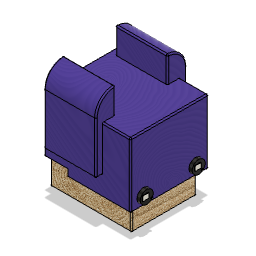
mouth 003 (Autodesk Fusion 360 design; units mm, degrees)
Autodesk Fusion 360 part; units mm, degrees
sketch "Sketch1" plane through (0, 0, 0) normal (0, 0, 1) x (1, 0, 0)
  line L0 (-50.4531, 15) -> (15, 15)
  line L1 (15, 15) -> (15, -10)
  line L2 (15, -10) -> (74.8522, -10)
  line L3 (74.8522, -10) -> (74.8522, -45)
  line L4 (74.8522, -45) -> (-50.4531, -45)
  line L5 (-50.4531, -45) -> (-50.4531, 15)
  constraint horizontal L0
  constraint perpendicular L0 L1
  constraint perpendicular L1 L2
  constraint perpendicular L2 L3
  constraint perpendicular L3 L4
  constraint perpendicular L0 L5
extrude "Extrude1" add sketch "Sketch1" along normal mid plane 100 makes body 1
shell "Shell1" thickness 5 removed faces 3 at (-6.8177, 15, 16.6667) at (15, 6.6667, -16.6667) at (34.9507, -10, -16.6667) on bodies 1
sketch "Sketch2" plane through (0, 0, 0) normal (0, 0, 1) x (1, 0, 0)
  circle A0 centre (0, 0) radius 5
  circle A1 centre (-39.3873, 8.5345) radius 5
  dimension "d4" = 10
  dimension "d5" = 10
  constraint coincident A0.centre origin
  measures "d4" diameter of A0
  measures "d5" diameter of A1
extrude "Extrude2" cut sketch "Sketch2" along normal mid plane 128 bodies 1
sketch "Sketch3" plane through (0, 0, 0) normal (0, 0, 1) x (1, 0, 0)
  line L0 (-50, 90) -> (-50, 0)
  line L1 (-50, 0) -> (-15, 0)
  line L2 (-15, -10) -> (83.2998, -10)
  line L3 (83.2998, -10) -> (83.2998, 90)
  line L4 (83.2998, 90) -> (-50, 90)
  line L5 (-15, 0) -> (-50, 0)
  line L6 (-15, 0) -> (-15, -10)
  constraint vertical L0
  constraint perpendicular L0 L1
  constraint perpendicular L0 L2
  constraint perpendicular L2 L3
  constraint perpendicular L0 L4
  constraint perpendicular L2 L6
extrude "Extrude3" add sketch "Sketch3" along normal mid plane 120 separate body makes body 2
sketch "Sketch4" plane through (-50, 0, 0) normal (-1, 0, 0) x (0, 0, 1)
  line L0 (-60, 0) -> (60, 0)
  line L1 (60, 0) -> (60, 90)
  line L2 (60, 90) -> (-60, 90)
  line L3 (-60, 90) -> (-60, 0)
  line L4 (50, -15) -> (-50, -15)
  line L5 (-50, -15) -> (-50, 20)
  line L6 (-50, 20) -> (50, 20)
  line L7 (50, 20) -> (50, -15)
  constraint horizontal L4
  constraint vertical L5
  constraint horizontal L6
  constraint vertical L7
extrude "Extrude4" cut sketch "Sketch4" against normal blind 120 contours L0 L5 L6 L7 | L0 L4 L5 L7 bodies 2
sketch "Sketch5" plane through (0, 0, 0) normal (0, 0, 1) x (1, 0, 0)
  circle A0 centre (0, 0) radius 5
  circle A1 centre (-39.3873, 8.5345) radius 5
  line L0 (-50.4531, -45) -> (74.8522, -45)
  line L1 (74.8522, -45) -> (74.8522, -10)
  line L2 (74.8522, -10) -> (15, -10)
  line L3 (15, -10) -> (15, 15)
  line L4 (15, 15) -> (-50.4531, 15)
  line L5 (-50.4531, 15) -> (-50.4531, -45)
extrude "Extrude5" add sketch "Sketch5" along normal mid plane 110 contours A1 bodies 2
sketch "Sketch6" plane through (0, 0, 0) normal (0, 0, 1) x (1, 0, 0)
  circle A0 centre (0, 0) radius 5
  circle A1 centre (-39.3873, 8.5345) radius 5
  line L0 (-50.4531, -45) -> (74.8522, -45)
  line L1 (74.8522, -45) -> (74.8522, -10)
  line L2 (74.8522, -10) -> (15, -10)
  line L3 (15, -10) -> (15, 15)
  line L4 (15, 15) -> (-50.4531, 15)
  line L5 (-50.4531, 15) -> (-50.4531, -45)
extrude "Extrude6" add sketch "Sketch6" along normal mid plane 100 separate body contours A0 makes body 3
sketch "Sketch8" plane through (0, 0, 0) normal (0, 0, 1) x (1, 0, 0)
  spline S0 degree 5 poles (0, 10) (-0.4483, 9.945) (-1.2891, 9.7827) (-2.3901, 9.3882) (-3.6145, 8.5811) (-5.0418, 7.1559) (-6.6425, 5.3776) (-8.5424, 3.3303) (-10.5598, 1.1324) (-12.3082, -1.0821) (-13.3437, -3.1875) (-13.2965, -5.0888) (-12.0101, -6.7454) (-9.6761, -8.1935) (-6.7064, -9.5182) (-3.614, -10.8275) (-0.8849, -12.2244) (1.132, -13.782) (2.3779, -15.5123) (3.0801, -17.3558) (3.5942, -19.1894) (4.2991, -20.8317) (5.4495, -22.0404) (7.1257, -22.5462) (9.2752, -22.1244) (11.7289, -20.6623) (14.2302, -18.2134) (16.4761, -14.9495) (18.1594, -11.1255) (19.0092, -7.0404) (18.8343, -2.999) (17.5607, 0.7235) (15.286, 3.9257) (12.2747, 6.494) (8.8775, 8.3796) (5.4706, 9.5855) (3.0039, 10.0369) (1.4007, 10.1128) (0.4483, 10.055) (0, 10) knots 0 0 0 0 0 0 0.028571 0.057143 0.085714 0.114286 0.142857 0.171429 0.2 0.228571 0.257143 0.285714 0.314286 0.342857 0.371429 0.4 0.428571 0.457143 0.485714 0.514286 0.542857 0.571429 0.6 0.628571 0.657143 0.685714 0.714286 0.742857 0.771429 0.8 0.828571 0.857143 0.885714 0.914286 0.942857 0.971429 1 1 1 1 1 1
  point P0 (-7, 5)
  point P1 (-13, -5)
  point P2 (0, -13)
  point P3 (4, -20)
  point P4 (9, -22)
  point P5 (18, -1)
extrude "Extrude8" add sketch "Sketch8" along normal mid plane 88 bodies 3
sketch "Sketch9" plane through (83.2998, 0, 0) normal (1, 0, 0) x (0, 0, -1)
  line L0 (60, 90) -> (-60, 90)
  line L1 (-60, 90) -> (-60, -10)
  line L2 (-60, -10) -> (60, -10)
  line L3 (60, -10) -> (60, 90)
  circle A0 centre (-40, 5) radius 10
  circle A1 centre (40, 5) radius 10
  dimension "d20" = 20
  dimension "d21" = 20
  measures "d20" diameter of A0
  measures "d21" diameter of A1
extrude "Extrude9" add sketch "Sketch9" along normal blind 5 contours A0 | A1 bodies 2
sketch "Sketch10" plane through (88.2998, 0, 0) normal (1, 0, 0) x (0, 0, -1)
  circle A0 centre (-40, 5) radius 10
  line L0 (-47.0368, 10.1033) -> (-37.5148, 10.1033)
  line L1 (-37.5148, 10.1033) -> (-37.5148, 2.6033)
  line L2 (-37.5148, 2.6033) -> (-47.0368, 2.6033)
  line L3 (-47.0368, 2.6033) -> (-47.0368, 10.1033)
  line L4 (-33.8726, 1.1981) -> (-31.8726, 1.1981)
  line L5 (-31.8726, 1.1981) -> (-31.8726, -0.8019)
  line L6 (-31.8726, -0.8019) -> (-33.8726, -0.8019)
  line L7 (-33.8726, -0.8019) -> (-33.8726, 1.1981)
  line L8 (33.4344, 10.1118) -> (42.9374, 10.1118)
  line L9 (42.9374, 10.1118) -> (42.9374, 2.6118)
  line L10 (42.9374, 2.6118) -> (33.4344, 2.6118)
  line L11 (33.4344, 2.6118) -> (33.4344, 10.1118)
  line L12 (44, 0) -> (46, 0)
  line L13 (46, 0) -> (46, -2)
  line L14 (46, -2) -> (44, -2)
  line L15 (44, -2) -> (44, 0)
  dimension "d24" = 9.522
  dimension "d25" = 7.5
  dimension "d26" = 2
  dimension "d27" = 2
  dimension "d28" = 9.503
  dimension "d29" = 7.5
  constraint horizontal L0
  constraint vertical L1
  constraint horizontal L2
  constraint vertical L3
  constraint horizontal L4
  constraint vertical L5
  constraint horizontal L6
  constraint vertical L7
  constraint horizontal L8
  constraint vertical L9
  constraint horizontal L10
  constraint vertical L11
  constraint horizontal L12
  constraint vertical L13
  constraint horizontal L14
  constraint vertical L15
  measures "d24" distance of L0.start L0.end
  measures "d25" distance of L0.start L2.end
  measures "d26" distance of L4.start L4.end
  measures "d27" distance of L4.start L6.end
  measures "d28" distance of L8.start L8.end
  measures "d29" distance of L8.start L10.end
extrude "Extrude10" add sketch "Sketch10" along normal blind 1 contours L0 L1 L2 L3 | L4 L5 L6 L7 | L8 L9 L10 L11 | L12 L13 L14 L15 bodies 2
fillet "Fillet1" radius 2 17 edges at (-50, 90, 0) (-50, 45, 60) (16.6499, 90, 60) (16.6499, 90, -60) (83.2998, 90, 0) (83.2998, 40, 60) (83.2998, 40, -60) (83.2998, -10, 0) (34.1499, -10, 60) (-15, -5, 60) (-32.5, 0, 60) (34.1499, -10, -60) (-15, -5, -60) (-32.5, 0, -60) (-50, 45, -60) (-50, 0, 55) (-15, 0, -55) on bodies 2
fillet "Fillet2" radius 2 9 edges at (74.8522, -27.5, -50) (74.8522, -45, 0) (74.8522, -27.5, 50) (12.1995, -45, -50) (12.1995, -45, 50) (-50.4531, -15, 50) (-50.4531, -45, 0) (-50.4531, -15, -50) (-50.4531, 15, 0) on bodies 1
sketch "Sketch11" plane through (0, 0, 0) normal (1, 0, 0) x (0, 0, -1)
  line L0 (-70, 130) -> (-40, 130)
  line L1 (-40, 130) -> (-40, 20)
  line L2 (-40, 20) -> (-70, 20)
  line L3 (-70, 20) -> (-70, 130)
  dimension "d36" = 30
  dimension "d37" = 110
  constraint horizontal L0
  constraint vertical L1
  constraint horizontal L2
  constraint vertical L3
  measures "d36" distance of L0.start L0.end
  measures "d37" distance of L0.start L2.end
extrude "Extrude11" add sketch "Sketch11" along normal mid plane 80 bodies 2
fillet "Fillet3" radius 30 1 edges at (0, 130, 70) on bodies 2
fillet "Fillet4" radius 2 10 edges at (0, 130, 40) (40, 60, 70) (40, 121.2132, 61.2132) (-40, 121.2132, 61.2132) (-40, 60, 70) (0, 20, 70) (40, 20, 65) (-40, 20, 65) (40, 110, 40) (-40, 110, 40) on bodies 2
mirror "Mirror1" about plane through (0, 0, 0) normal (0, 0, 1) of "Extrude11", "Fillet3", "Fillet4"
